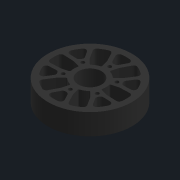
# Autodesk Inventor part: 4 inch 60a - 1 thick
Saved by Autodesk Inventor 2021 (Build 250183000, 183)
## iProperties
Created: 2018-05-25
Part Number: 4 inch 60a - 1 thick
Material: Generic
Description: STEP AP214
Document SubType Name: Modeling
Designer: max
Density: 1 g/cm^3
Appearance: 60a Flex Wheel
Sending System: SolidWorks 2017
Preprocessor: SwSTEP 2.0
Title: 217-6450-20180525.STEP
Revision Number: ANY
Autodesk Inventor part; units mm, degrees
ref_plane "YZ Plane" through (0, 0, 0) normal (1, 0, 0) x (0, 1, 0)
ref_plane "XZ Plane" through (0, 0, 0) normal (0, 1, 0) x (-1, 0, 0)
ref_plane "XY Plane" through (0, 0, 0) normal (0, 0, 1) x (1, 0, 0)
sketch "Sketch1" plane through (0, 12.7, 0) normal (0, 1, 0) x (1, 0, 0)
  circle A0 centre (0, 0) radius 50.8 projected
  circle A1 centre (0, 0) radius 14 projected
  line L0 (24.8683, -18.6819) -> (29.4395, -25.8574) projected
  arc A2 (24.8242, -14.992) -> (24.8683, -18.6819) centre (27.8202, -16.8014) ccw projected
  arc A3 (24.8242, -14.992) -> (25.3956, -14.0023) centre (0, 0) ccw projected
  arc A4 (28.6132, -12.1956) -> (25.3956, -14.0023) centre (28.4605, -15.6923) ccw projected
  line L1 (37.1129, -12.5666) -> (28.6132, -12.1956) projected
  arc A5 (40.1702, -17.4584) -> (37.1129, -12.5666) centre (36.9603, -16.0633) ccw projected
  arc A6 (35.2045, -26.0592) -> (40.1702, -17.4584) centre (0, 0) ccw projected
  arc A7 (29.4395, -25.8574) -> (35.2045, -26.0592) centre (32.3914, -23.9769) ccw projected
  arc A8 (5.8117, -18.6138) -> (13.2142, -14.34) centre (0, 0) ccw projected
  arc A9 (14.599, -14.3683) -> (13.2142, -14.34) centre (13.8918, -15.0754) ccw projected
  line L2 (20.3501, -20.1194) -> (14.599, -14.3683) projected
  arc A10 (20.8271, -20.7137) -> (20.3501, -20.1194) centre (17.8752, -22.5942) ccw projected
  line L3 (27.0236, -30.4404) -> (20.8271, -20.7137) projected
  arc A11 (26.1623, -35.128) -> (27.0236, -30.4404) centre (24.0717, -32.321) ccw projected
  arc A12 (17.3406, -40.2212) -> (26.1623, -35.128) centre (0, 0) ccw projected
  arc A13 (12.8504, -38.6233) -> (17.3406, -40.2212) centre (15.9549, -37.0072) ccw projected
  line L4 (7.5251, -28.3936) -> (12.8504, -38.6233) projected
  arc A14 (7.2489, -27.6834) -> (7.5251, -28.3936) centre (10.6296, -26.7775) ccw projected
  line L5 (5.1438, -19.8272) -> (7.2489, -27.6834) projected
  arc A15 (5.8117, -18.6138) -> (5.1438, -19.8272) centre (6.1097, -19.5684) ccw projected
  line L6 (-3.7449, -30.8775) -> (-7.6734, -38.424) projected
  arc A16 (-0.5714, -28.9944) -> (-3.7449, -30.8775) centre (-0.6404, -32.4937) ccw projected
  arc A17 (-0.5714, -28.9944) -> (0.5714, -28.9944) centre (0, 0) ccw projected
  arc A18 (3.7449, -30.8775) -> (0.5714, -28.9944) centre (0.6404, -32.4937) ccw projected
  line L7 (7.6734, -38.424) -> (3.7449, -30.8775) projected
  arc A19 (4.9657, -43.5176) -> (7.6734, -38.424) centre (4.5689, -40.0402) ccw projected
  arc A20 (-4.9657, -43.5176) -> (4.9657, -43.5176) centre (0, 0) ccw projected
  arc A21 (-7.6734, -38.424) -> (-4.9657, -43.5176) centre (-4.5689, -40.0402) ccw projected
  arc A22 (-13.2142, -14.34) -> (-5.8117, -18.6138) centre (0, 0) ccw projected
  arc A23 (-5.1438, -19.8272) -> (-5.8117, -18.6138) centre (-6.1097, -19.5684) ccw projected
  line L8 (-7.2489, -27.6834) -> (-5.1438, -19.8272) projected
  arc A24 (-7.5251, -28.3936) -> (-7.2489, -27.6834) centre (-10.6296, -26.7775) ccw projected
  line L9 (-12.8504, -38.6233) -> (-7.5251, -28.3936) projected
  arc A25 (-17.3406, -40.2212) -> (-12.8504, -38.6233) centre (-15.9549, -37.0072) ccw projected
  arc A26 (-26.1623, -35.128) -> (-17.3406, -40.2212) centre (0, 0) ccw projected
  arc A27 (-27.0236, -30.4404) -> (-26.1623, -35.128) centre (-24.0717, -32.321) ccw projected
  line L10 (-20.8271, -20.7137) -> (-27.0236, -30.4404) projected
  arc A28 (-20.3501, -20.1194) -> (-20.8271, -20.7137) centre (-17.8752, -22.5942) ccw projected
  line L11 (-14.599, -14.3683) -> (-20.3501, -20.1194) projected
  arc A29 (-13.2142, -14.34) -> (-14.599, -14.3683) centre (-13.8918, -15.0754) ccw projected
  arc A30 (-24.8242, 14.992) -> (-25.3956, 14.0023) centre (0, 0) ccw projected
  arc A31 (-28.6132, 12.1956) -> (-25.3956, 14.0023) centre (-28.4605, 15.6923) ccw projected
  line L12 (-37.1129, 12.5666) -> (-28.6132, 12.1956) projected
  arc A32 (-40.1702, 17.4584) -> (-37.1129, 12.5666) centre (-36.9603, 16.0633) ccw projected
  arc A33 (-35.2045, 26.0592) -> (-40.1702, 17.4584) centre (0, 0) ccw projected
  arc A34 (-29.4395, 25.8574) -> (-35.2045, 26.0592) centre (-32.3914, 23.9769) ccw projected
  line L13 (-24.8683, 18.6819) -> (-29.4395, 25.8574) projected
  arc A35 (-24.8242, 14.992) -> (-24.8683, 18.6819) centre (-27.8202, 16.8014) ccw projected
  arc A36 (-19.0259, 4.2738) -> (-19.0259, -4.2738) centre (0, 0) ccw projected
  arc A37 (-19.7428, -5.4589) -> (-19.0259, -4.2738) centre (-20.0016, -4.493) ccw projected
  line L14 (-27.5989, -7.564) -> (-19.7428, -5.4589) projected
  arc A38 (-28.3521, -7.6799) -> (-27.5989, -7.564) centre (-28.5048, -4.1833) ccw projected
  line L15 (-39.874, -8.1829) -> (-28.3521, -7.6799) projected
  arc A39 (-43.5029, -5.0932) -> (-39.874, -8.1829) centre (-40.0266, -4.6862) ccw projected
  arc A40 (-43.5029, 5.0932) -> (-43.5029, -5.0932) centre (0, 0) ccw projected
  arc A41 (-39.874, 8.1829) -> (-43.5029, 5.0932) centre (-40.0266, 4.6862) ccw projected
  line L16 (-28.3521, 7.6799) -> (-39.874, 8.1829) projected
  arc A42 (-27.5989, 7.564) -> (-28.3521, 7.6799) centre (-28.5048, 4.1833) ccw projected
  line L17 (-19.7428, 5.4589) -> (-27.5989, 7.564) projected
  arc A43 (-19.0259, 4.2738) -> (-19.7428, 5.4589) centre (-20.0016, 4.493) ccw projected
  arc A44 (13.2142, 14.34) -> (5.8117, 18.6138) centre (0, 0) ccw projected
  arc A45 (5.1438, 19.8272) -> (5.8117, 18.6138) centre (6.1097, 19.5684) ccw projected
  line L18 (7.2489, 27.6834) -> (5.1438, 19.8272) projected
  arc A46 (7.5251, 28.3936) -> (7.2489, 27.6834) centre (10.6296, 26.7775) ccw projected
  line L19 (12.8504, 38.6233) -> (7.5251, 28.3936) projected
  arc A47 (17.3406, 40.2212) -> (12.8504, 38.6233) centre (15.9549, 37.0072) ccw projected
  arc A48 (26.1623, 35.128) -> (17.3406, 40.2212) centre (0, 0) ccw projected
  arc A49 (27.0236, 30.4404) -> (26.1623, 35.128) centre (24.0717, 32.321) ccw projected
  line L20 (20.8271, 20.7137) -> (27.0236, 30.4404) projected
  arc A50 (20.3501, 20.1194) -> (20.8271, 20.7137) centre (17.8752, 22.5942) ccw projected
  line L21 (14.599, 14.3683) -> (20.3501, 20.1194) projected
  arc A51 (13.2142, 14.34) -> (14.599, 14.3683) centre (13.8918, 15.0754) ccw projected
  line L22 (28.6132, 12.1956) -> (37.1129, 12.5666) projected
  arc A52 (25.3956, 14.0023) -> (28.6132, 12.1956) centre (28.4605, 15.6923) ccw projected
  arc A53 (25.3956, 14.0023) -> (24.8242, 14.992) centre (0, 0) ccw projected
  arc A54 (24.8683, 18.6819) -> (24.8242, 14.992) centre (27.8202, 16.8014) ccw projected
  line L23 (29.4395, 25.8574) -> (24.8683, 18.6819) projected
  arc A55 (35.2045, 26.0592) -> (29.4395, 25.8574) centre (32.3914, 23.9769) ccw projected
  arc A56 (40.1702, 17.4584) -> (35.2045, 26.0592) centre (0, 0) ccw projected
  arc A57 (37.1129, 12.5666) -> (40.1702, 17.4584) centre (36.9603, 16.0633) ccw projected
  arc A58 (19.0259, -4.2738) -> (19.0259, 4.2738) centre (0, 0) ccw projected
  arc A59 (19.7428, 5.4589) -> (19.0259, 4.2738) centre (20.0016, 4.493) ccw projected
  line L24 (27.5989, 7.564) -> (19.7428, 5.4589) projected
  arc A60 (28.3521, 7.6799) -> (27.5989, 7.564) centre (28.5048, 4.1833) ccw projected
  line L25 (39.874, 8.1829) -> (28.3521, 7.6799) projected
  arc A61 (43.5029, 5.0932) -> (39.874, 8.1829) centre (40.0266, 4.6862) ccw projected
  arc A62 (43.5029, -5.0932) -> (43.5029, 5.0932) centre (0, 0) ccw projected
  arc A63 (39.874, -8.1829) -> (43.5029, -5.0932) centre (40.0266, -4.6862) ccw projected
  line L26 (28.3521, -7.6799) -> (39.874, -8.1829) projected
  arc A64 (27.5989, -7.564) -> (28.3521, -7.6799) centre (28.5048, -4.1833) ccw projected
  line L27 (19.7428, -5.4589) -> (27.5989, -7.564) projected
  arc A65 (19.0259, -4.2738) -> (19.7428, -5.4589) centre (20.0016, -4.493) ccw projected
  line L28 (3.7449, 30.8775) -> (7.6734, 38.424) projected
  arc A66 (0.5714, 28.9944) -> (3.7449, 30.8775) centre (0.6404, 32.4937) ccw projected
  arc A67 (0.5714, 28.9944) -> (-0.5714, 28.9944) centre (0, 0) ccw projected
  arc A68 (-3.7449, 30.8775) -> (-0.5714, 28.9944) centre (-0.6404, 32.4937) ccw projected
  line L29 (-7.6734, 38.424) -> (-3.7449, 30.8775) projected
  arc A69 (-4.9657, 43.5176) -> (-7.6734, 38.424) centre (-4.5689, 40.0402) ccw projected
  arc A70 (4.9657, 43.5176) -> (-4.9657, 43.5176) centre (0, 0) ccw projected
  arc A71 (7.6734, 38.424) -> (4.9657, 43.5176) centre (4.5689, 40.0402) ccw projected
  line L30 (-28.6132, -12.1956) -> (-37.1129, -12.5666) projected
  arc A72 (-25.3956, -14.0023) -> (-28.6132, -12.1956) centre (-28.4605, -15.6923) ccw projected
  arc A73 (-25.3956, -14.0023) -> (-24.8242, -14.992) centre (0, 0) ccw projected
  arc A74 (-24.8683, -18.6819) -> (-24.8242, -14.992) centre (-27.8202, -16.8014) ccw projected
  line L31 (-29.4395, -25.8574) -> (-24.8683, -18.6819) projected
  arc A75 (-35.2045, -26.0592) -> (-29.4395, -25.8574) centre (-32.3914, -23.9769) ccw projected
  arc A76 (-40.1702, -17.4584) -> (-35.2045, -26.0592) centre (0, 0) ccw projected
  arc A77 (-37.1129, -12.5666) -> (-40.1702, -17.4584) centre (-36.9603, -16.0633) ccw projected
  arc A78 (-5.8117, 18.6138) -> (-13.2142, 14.34) centre (0, 0) ccw projected
  arc A79 (-14.599, 14.3683) -> (-13.2142, 14.34) centre (-13.8918, 15.0754) ccw projected
  line L32 (-20.3501, 20.1194) -> (-14.599, 14.3683) projected
  arc A80 (-20.8271, 20.7137) -> (-20.3501, 20.1194) centre (-17.8752, 22.5942) ccw projected
  line L33 (-27.0236, 30.4404) -> (-20.8271, 20.7137) projected
  arc A81 (-26.1623, 35.128) -> (-27.0236, 30.4404) centre (-24.0717, 32.321) ccw projected
  arc A82 (-17.3406, 40.2212) -> (-26.1623, 35.128) centre (0, 0) ccw projected
  arc A83 (-12.8504, 38.6233) -> (-17.3406, 40.2212) centre (-15.9549, 37.0072) ccw projected
  line L34 (-7.5251, 28.3936) -> (-12.8504, 38.6233) projected
  arc A84 (-7.2489, 27.6834) -> (-7.5251, 28.3936) centre (-10.6296, 26.7775) ccw projected
  line L35 (-5.1438, 19.8272) -> (-7.2489, 27.6834) projected
  arc A85 (-5.8117, 18.6138) -> (-5.1438, 19.8272) centre (-6.1097, 19.5684) ccw projected
  circle A86 centre (20.6222, 11.9063) radius 2.1526 projected
  circle A87 centre (20.6222, -11.9062) radius 2.1526 projected
  circle A88 centre (0, -23.8125) radius 2.1526 projected
  circle A89 centre (-20.6222, -11.9063) radius 2.1526 projected
  circle A90 centre (-20.6222, 11.9062) radius 2.1526 projected
  circle A91 centre (0, 23.8125) radius 2.1526 projected
extrude "Extrusion1" add sketch "Sketch1" along normal blind 25.4
sketch "Sketch2" plane through (0, -12.7, 0) normal (0, -1, 0) x (1, 0, 0)
  circle A0 centre (0, 0) radius 50.8 projected
  circle A1 centre (0, 0) radius 14 projected
  line L0 (37.1129, 12.5666) -> (28.6132, 12.1956) projected
  arc A2 (25.3956, 14.0023) -> (28.6132, 12.1956) centre (28.4605, 15.6923) ccw projected
  arc A3 (25.3956, 14.0023) -> (24.8242, 14.992) centre (0, 0) ccw projected
  arc A4 (24.8683, 18.6819) -> (24.8242, 14.992) centre (27.8202, 16.8014) ccw projected
  line L1 (24.8683, 18.6819) -> (29.4395, 25.8574) projected
  arc A5 (35.2045, 26.0592) -> (29.4395, 25.8574) centre (32.3914, 23.9769) ccw projected
  arc A6 (40.1702, 17.4584) -> (35.2045, 26.0592) centre (0, 0) ccw projected
  arc A7 (37.1129, 12.5666) -> (40.1702, 17.4584) centre (36.9603, 16.0633) ccw projected
  line L2 (27.0236, 30.4404) -> (20.8271, 20.7137) projected
  arc A8 (20.3501, 20.1194) -> (20.8271, 20.7137) centre (17.8752, 22.5942) ccw projected
  line L3 (20.3501, 20.1194) -> (14.599, 14.3683) projected
  arc A9 (13.2142, 14.34) -> (14.599, 14.3683) centre (13.8918, 15.0754) ccw projected
  arc A10 (13.2142, 14.34) -> (5.8117, 18.6138) centre (0, 0) ccw projected
  arc A11 (5.1438, 19.8272) -> (5.8117, 18.6138) centre (6.1097, 19.5684) ccw projected
  line L4 (5.1438, 19.8272) -> (7.2489, 27.6834) projected
  arc A12 (7.5251, 28.3936) -> (7.2489, 27.6834) centre (10.6296, 26.7775) ccw projected
  line L5 (7.5251, 28.3936) -> (12.8504, 38.6233) projected
  arc A13 (17.3406, 40.2212) -> (12.8504, 38.6233) centre (15.9549, 37.0072) ccw projected
  arc A14 (26.1623, 35.128) -> (17.3406, 40.2212) centre (0, 0) ccw projected
  arc A15 (27.0236, 30.4404) -> (26.1623, 35.128) centre (24.0717, 32.321) ccw projected
  line L6 (7.6734, 38.424) -> (3.7449, 30.8775) projected
  arc A16 (0.5714, 28.9944) -> (3.7449, 30.8775) centre (0.6404, 32.4937) ccw projected
  arc A17 (0.5714, 28.9944) -> (-0.5714, 28.9944) centre (0, 0) ccw projected
  arc A18 (-3.7449, 30.8775) -> (-0.5714, 28.9944) centre (-0.6404, 32.4937) ccw projected
  line L7 (-3.7449, 30.8775) -> (-7.6734, 38.424) projected
  arc A19 (-4.9657, 43.5176) -> (-7.6734, 38.424) centre (-4.5689, 40.0402) ccw projected
  arc A20 (4.9657, 43.5176) -> (-4.9657, 43.5176) centre (0, 0) ccw projected
  arc A21 (7.6734, 38.424) -> (4.9657, 43.5176) centre (4.5689, 40.0402) ccw projected
  line L8 (-12.8504, 38.6233) -> (-7.5251, 28.3936) projected
  arc A22 (-7.2489, 27.6834) -> (-7.5251, 28.3936) centre (-10.6296, 26.7775) ccw projected
  line L9 (-7.2489, 27.6834) -> (-5.1438, 19.8272) projected
  arc A23 (-5.8117, 18.6138) -> (-5.1438, 19.8272) centre (-6.1097, 19.5684) ccw projected
  arc A24 (-5.8117, 18.6138) -> (-13.2142, 14.34) centre (0, 0) ccw projected
  arc A25 (-14.599, 14.3683) -> (-13.2142, 14.34) centre (-13.8918, 15.0754) ccw projected
  line L10 (-14.599, 14.3683) -> (-20.3501, 20.1194) projected
  arc A26 (-20.8271, 20.7137) -> (-20.3501, 20.1194) centre (-17.8752, 22.5942) ccw projected
  line L11 (-20.8271, 20.7137) -> (-27.0236, 30.4404) projected
  arc A27 (-26.1623, 35.128) -> (-27.0236, 30.4404) centre (-24.0717, 32.321) ccw projected
  arc A28 (-17.3406, 40.2212) -> (-26.1623, 35.128) centre (0, 0) ccw projected
  arc A29 (-12.8504, 38.6233) -> (-17.3406, 40.2212) centre (-15.9549, 37.0072) ccw projected
  line L12 (-39.874, 8.1829) -> (-28.3521, 7.6799) projected
  arc A30 (-27.5989, 7.564) -> (-28.3521, 7.6799) centre (-28.5048, 4.1833) ccw projected
  line L13 (-27.5989, 7.564) -> (-19.7428, 5.4589) projected
  arc A31 (-19.0259, 4.2738) -> (-19.7428, 5.4589) centre (-20.0016, 4.493) ccw projected
  arc A32 (-19.0259, 4.2738) -> (-19.0259, -4.2738) centre (0, 0) ccw projected
  arc A33 (-19.7428, -5.4589) -> (-19.0259, -4.2738) centre (-20.0016, -4.493) ccw projected
  line L14 (-19.7428, -5.4589) -> (-27.5989, -7.564) projected
  arc A34 (-28.3521, -7.6799) -> (-27.5989, -7.564) centre (-28.5048, -4.1833) ccw projected
  line L15 (-28.3521, -7.6799) -> (-39.874, -8.1829) projected
  arc A35 (-43.5029, -5.0932) -> (-39.874, -8.1829) centre (-40.0266, -4.6862) ccw projected
  arc A36 (-43.5029, 5.0932) -> (-43.5029, -5.0932) centre (0, 0) ccw projected
  arc A37 (-39.874, 8.1829) -> (-43.5029, 5.0932) centre (-40.0266, 4.6862) ccw projected
  line L16 (12.8504, -38.6233) -> (7.5251, -28.3936) projected
  arc A38 (7.2489, -27.6834) -> (7.5251, -28.3936) centre (10.6296, -26.7775) ccw projected
  line L17 (7.2489, -27.6834) -> (5.1438, -19.8272) projected
  arc A39 (5.8117, -18.6138) -> (5.1438, -19.8272) centre (6.1097, -19.5684) ccw projected
  arc A40 (5.8117, -18.6138) -> (13.2142, -14.34) centre (0, 0) ccw projected
  arc A41 (14.599, -14.3683) -> (13.2142, -14.34) centre (13.8918, -15.0754) ccw projected
  line L18 (14.599, -14.3683) -> (20.3501, -20.1194) projected
  arc A42 (20.8271, -20.7137) -> (20.3501, -20.1194) centre (17.8752, -22.5942) ccw projected
  line L19 (20.8271, -20.7137) -> (27.0236, -30.4404) projected
  arc A43 (26.1623, -35.128) -> (27.0236, -30.4404) centre (24.0717, -32.321) ccw projected
  arc A44 (17.3406, -40.2212) -> (26.1623, -35.128) centre (0, 0) ccw projected
  arc A45 (12.8504, -38.6233) -> (17.3406, -40.2212) centre (15.9549, -37.0072) ccw projected
  line L20 (29.4395, -25.8574) -> (24.8683, -18.6819) projected
  arc A46 (24.8242, -14.992) -> (24.8683, -18.6819) centre (27.8202, -16.8014) ccw projected
  arc A47 (24.8242, -14.992) -> (25.3956, -14.0023) centre (0, 0) ccw projected
  arc A48 (28.6132, -12.1956) -> (25.3956, -14.0023) centre (28.4605, -15.6923) ccw projected
  line L21 (28.6132, -12.1956) -> (37.1129, -12.5666) projected
  arc A49 (40.1702, -17.4584) -> (37.1129, -12.5666) centre (36.9603, -16.0633) ccw projected
  arc A50 (35.2045, -26.0592) -> (40.1702, -17.4584) centre (0, 0) ccw projected
  arc A51 (29.4395, -25.8574) -> (35.2045, -26.0592) centre (32.3914, -23.9769) ccw projected
  line L22 (39.874, -8.1829) -> (28.3521, -7.6799) projected
  arc A52 (27.5989, -7.564) -> (28.3521, -7.6799) centre (28.5048, -4.1833) ccw projected
  line L23 (27.5989, -7.564) -> (19.7428, -5.4589) projected
  arc A53 (19.0259, -4.2738) -> (19.7428, -5.4589) centre (20.0016, -4.493) ccw projected
  arc A54 (19.0259, -4.2738) -> (19.0259, 4.2738) centre (0, 0) ccw projected
  arc A55 (19.7428, 5.4589) -> (19.0259, 4.2738) centre (20.0016, 4.493) ccw projected
  line L24 (19.7428, 5.4589) -> (27.5989, 7.564) projected
  arc A56 (28.3521, 7.6799) -> (27.5989, 7.564) centre (28.5048, 4.1833) ccw projected
  line L25 (28.3521, 7.6799) -> (39.874, 8.1829) projected
  arc A57 (43.5029, 5.0932) -> (39.874, 8.1829) centre (40.0266, 4.6862) ccw projected
  arc A58 (43.5029, -5.0932) -> (43.5029, 5.0932) centre (0, 0) ccw projected
  arc A59 (39.874, -8.1829) -> (43.5029, -5.0932) centre (40.0266, -4.6862) ccw projected
  arc A60 (-0.5714, -28.9944) -> (0.5714, -28.9944) centre (0, 0) ccw projected
  arc A61 (3.7449, -30.8775) -> (0.5714, -28.9944) centre (0.6404, -32.4937) ccw projected
  line L26 (3.7449, -30.8775) -> (7.6734, -38.424) projected
  arc A62 (4.9657, -43.5176) -> (7.6734, -38.424) centre (4.5689, -40.0402) ccw projected
  arc A63 (-4.9657, -43.5176) -> (4.9657, -43.5176) centre (0, 0) ccw projected
  arc A64 (-7.6734, -38.424) -> (-4.9657, -43.5176) centre (-4.5689, -40.0402) ccw projected
  line L27 (-7.6734, -38.424) -> (-3.7449, -30.8775) projected
  arc A65 (-0.5714, -28.9944) -> (-3.7449, -30.8775) centre (-0.6404, -32.4937) ccw projected
  line L28 (-29.4395, 25.8574) -> (-24.8683, 18.6819) projected
  arc A66 (-24.8242, 14.992) -> (-24.8683, 18.6819) centre (-27.8202, 16.8014) ccw projected
  arc A67 (-24.8242, 14.992) -> (-25.3956, 14.0023) centre (0, 0) ccw projected
  arc A68 (-28.6132, 12.1956) -> (-25.3956, 14.0023) centre (-28.4605, 15.6923) ccw projected
  line L29 (-28.6132, 12.1956) -> (-37.1129, 12.5666) projected
  arc A69 (-40.1702, 17.4584) -> (-37.1129, 12.5666) centre (-36.9603, 16.0633) ccw projected
  arc A70 (-35.2045, 26.0592) -> (-40.1702, 17.4584) centre (0, 0) ccw projected
  arc A71 (-29.4395, 25.8574) -> (-35.2045, 26.0592) centre (-32.3914, 23.9769) ccw projected
  line L30 (-27.0236, -30.4404) -> (-20.8271, -20.7137) projected
  arc A72 (-20.3501, -20.1194) -> (-20.8271, -20.7137) centre (-17.8752, -22.5942) ccw projected
  line L31 (-20.3501, -20.1194) -> (-14.599, -14.3683) projected
  arc A73 (-13.2142, -14.34) -> (-14.599, -14.3683) centre (-13.8918, -15.0754) ccw projected
  arc A74 (-13.2142, -14.34) -> (-5.8117, -18.6138) centre (0, 0) ccw projected
  arc A75 (-5.1438, -19.8272) -> (-5.8117, -18.6138) centre (-6.1097, -19.5684) ccw projected
  line L32 (-5.1438, -19.8272) -> (-7.2489, -27.6834) projected
  arc A76 (-7.5251, -28.3936) -> (-7.2489, -27.6834) centre (-10.6296, -26.7775) ccw projected
  line L33 (-7.5251, -28.3936) -> (-12.8504, -38.6233) projected
  arc A77 (-17.3406, -40.2212) -> (-12.8504, -38.6233) centre (-15.9549, -37.0072) ccw projected
  arc A78 (-26.1623, -35.128) -> (-17.3406, -40.2212) centre (0, 0) ccw projected
  arc A79 (-27.0236, -30.4404) -> (-26.1623, -35.128) centre (-24.0717, -32.321) ccw projected
  arc A80 (-40.1702, -17.4584) -> (-35.2045, -26.0592) centre (0, 0) ccw projected
  arc A81 (-37.1129, -12.5666) -> (-40.1702, -17.4584) centre (-36.9603, -16.0633) ccw projected
  line L34 (-37.1129, -12.5666) -> (-28.6132, -12.1956) projected
  arc A82 (-25.3956, -14.0023) -> (-28.6132, -12.1956) centre (-28.4605, -15.6923) ccw projected
  arc A83 (-25.3956, -14.0023) -> (-24.8242, -14.992) centre (0, 0) ccw projected
  arc A84 (-24.8683, -18.6819) -> (-24.8242, -14.992) centre (-27.8202, -16.8014) ccw projected
  line L35 (-24.8683, -18.6819) -> (-29.4395, -25.8574) projected
  arc A85 (-35.2045, -26.0592) -> (-29.4395, -25.8574) centre (-32.3914, -23.9769) ccw projected
  circle A86 centre (20.6222, -11.9063) radius 2.1526 projected
  circle A87 centre (20.6222, 11.9062) radius 2.1526 projected
  circle A88 centre (0, 23.8125) radius 2.1526 projected
  circle A89 centre (-20.6222, 11.9063) radius 2.1526 projected
  circle A90 centre (-20.6222, -11.9062) radius 2.1526 projected
  circle A91 centre (0, -23.8125) radius 2.1526 projected
extrude "Extrusion2" cut sketch "Sketch2" against normal blind 25.4
body "Solid1"
